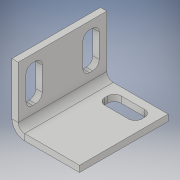
# Autodesk Inventor part: mezzanineBracketRight
Saved by Autodesk Inventor 2017 (Build 210142000, 142)
## iProperties
Created: 2017-03-16
Part Number: mezzanineBracketRight
Material: Generic
Document SubType Name: Sheet Metal
Designer: Zara
Density: 1 g/cm^3
Sheet Metal Rule: Default
Appearance: Default
Author: Zara
Autodesk Inventor part; units mm, degrees
ref_plane "YZ Plane" through (0, 0, 0) normal (1, 0, 0) x (0, 1, 0)
ref_plane "XZ Plane" through (0, 0, 0) normal (0, 1, 0) x (-1, 0, 0)
ref_plane "XY Plane" through (0, 0, 0) normal (0, 0, 1) x (1, 0, 0)
sketch "Sketch1" plane through (0, 0, 0) normal (0, 1, 0) x (-1, 0, 0)
  line L0 (-8.128, 10.6426) -> (8.128, 10.6426)
  line L1 (8.128, 10.6426) -> (8.128, -10.6426)
  line L2 (8.128, -10.6426) -> (-8.128, -10.6426)
  line L3 (-8.128, -10.6426) -> (-8.128, 10.6426)
  line L4 (-8.128, 10.6426) -> (8.128, -10.6426) construction
  line L5 (8.128, 10.6426) -> (-8.128, -10.6426) construction
  point P0 (0, 0)
  dimension "d0" = 21.2852
  dimension "d1" = 16.256
  measures "d0" distance of L0.end L1.end
  measures "d1" distance of L1.end L2.end
extrude "Plate1" add sketch "Sketch1" along normal blind 1.524
sketch "Sketch2" plane through (-6.604, 0, 10.6426) normal (-1, 0, 0) x (0, -1, 0)
  line L0 (0, -21.2852) -> (0, 0)
  line L1 (0, 0) -> (-15.5956, 0)
  line L2 (-15.5956, 0) -> (-15.5956, -21.2852)
  line L3 (-15.5956, -21.2852) -> (0, -21.2852)
  constraints: 6 end point, 1 horizontal, 1 perpendicular, 1 vertical
edge flange "Flange1" height 15.5956 angle 90 thickness 1.524 bend radius 1.524 thickness toward (-1, 0, 0) relief tear relief width 1.524 relief depth 0.762 edges at (-8.128, 1.524, 0) wall of the first edge with corners at (-6.604, 0, -10.6426) (-6.604, 0, 10.6426) (-6.604, 15.5956, 10.6426) (-6.604, 15.5956, -10.6426)
bend "Bend1"
corner "Corner1"
sketch "Sketch3" plane through (-6.604, 15.5956, 10.6426) normal (1, 0, 0) x (0, 0, -1)
  line L0 (0, 0) -> (0, -12.5476) construction
  line L1 (21.2852, -12.5476) -> (21.2852, 0) construction
  circle A0 centre (3.7973, -6.2738) radius 1.5875 construction
  circle A1 centre (17.4879, -6.2738) radius 1.5875 construction
  line L2 (3.7973, -6.2738) -> (17.4879, -6.2738) construction
  line L3 (21.2852, 0) -> (0, 0) construction
  line L4 (10.6426, 0) -> (10.6426, -12.5476) construction
  line L5 (0, -12.5476) -> (21.2852, -12.5476) construction
  line L6 (17.1196, -10.7188) -> (17.8562, -10.7188)
  line L7 (19.4437, -9.1313) -> (19.4437, -3.4163)
  line L8 (17.8562, -1.8288) -> (17.1196, -1.8288)
  line L9 (15.5321, -3.4163) -> (15.5321, -9.1313)
  line L10 (15.5321, -10.7188) -> (19.4437, -1.8288) construction
  line L11 (19.4437, -10.7188) -> (15.5321, -1.8288) construction
  arc A2 (17.1196, -1.8288) -> (15.5321, -3.4163) centre (17.1196, -3.4163) ccw
  arc A3 (19.4437, -3.4163) -> (17.8562, -1.8288) centre (17.8562, -3.4163) ccw
  arc A4 (15.5321, -9.1313) -> (17.1196, -10.7188) centre (17.1196, -9.1313) ccw
  arc A5 (17.8562, -10.7188) -> (19.4437, -9.1313) centre (17.8562, -9.1313) ccw
  line L12 (3.429, -10.7188) -> (4.1656, -10.7188)
  line L13 (5.7531, -9.1313) -> (5.7531, -3.4163)
  line L14 (4.1656, -1.8288) -> (3.429, -1.8288)
  line L15 (1.8415, -3.4163) -> (1.8415, -9.1313)
  line L16 (1.8415, -10.7188) -> (5.7531, -1.8288) construction
  line L17 (5.7531, -10.7188) -> (1.8415, -1.8288) construction
  arc A6 (3.429, -1.8288) -> (1.8415, -3.4163) centre (3.429, -3.4163) ccw
  arc A7 (5.7531, -3.4163) -> (4.1656, -1.8288) centre (4.1656, -3.4163) ccw
  arc A8 (4.1656, -10.7188) -> (5.7531, -9.1313) centre (4.1656, -9.1313) ccw
  arc A9 (1.8415, -9.1313) -> (3.429, -10.7188) centre (3.429, -9.1313) ccw
  point P0 (10.6426, -15.5956)
  point P1 (10.6426, -6.2738)
  dimension "d13" = 13.6906
  dimension "d14" = 3.175
  dimension "d15" = 3.175
  dimension "d16" = 3.9116
  dimension "d17" = 8.89
  dimension "d18" = 1.5875
  dimension "d19" = 3.9116
  dimension "d20" = 8.89
  dimension "d21" = 1.5875
  constraints: 28 end point, 16 point on circle, 16 point on line, 16 tangent, 10 centre point, 8 midpoint, 6 equal radius, 4 parallel, 3 horizontal, 2 perpendicular
  measures "d13" distance of L2.end L2.start
  measures "d14" diameter of A1
  measures "d15" diameter of A0
  measures "d16" distance of L10.start L11.start
  measures "d17" distance of L11.start L10.end
  measures "d18" radius of A2
  measures "d19" distance of L16.start L17.start
  measures "d20" distance of L17.end L16.start
  measures "d21" radius of A6
sketch "Sketch4" plane through (0, 1.524, 0) normal (0, 1, 0) x (1, 0, 0)
  line L0 (-5.08, 10.6426) -> (8.128, 10.6426) construction
  line L1 (4.3815, 4.8768) -> (-1.3335, 4.8768)
  line L2 (-2.921, 6.4643) -> (-2.921, 7.2009)
  line L3 (-1.3335, 8.7884) -> (4.3815, 8.7884)
  line L4 (5.969, 7.2009) -> (5.969, 6.4643)
  arc A0 (-2.921, 6.4643) -> (-1.3335, 4.8768) centre (-1.3335, 6.4643) ccw
  arc A1 (-1.3335, 8.7884) -> (-2.921, 7.2009) centre (-1.3335, 7.2009) ccw
  arc A2 (4.3815, 4.8768) -> (5.969, 6.4643) centre (4.3815, 6.4643) ccw
  arc A3 (5.969, 7.2009) -> (4.3815, 8.7884) centre (4.3815, 7.2009) ccw
  line L5 (8.128, 10.6426) -> (8.128, -10.6426) projected
  line L6 (1.524, 4.8768) -> (1.524, 8.7884) construction
  line L7 (4.3815, -8.7884) -> (-1.3335, -8.7884) construction
  line L8 (-2.921, -7.2009) -> (-2.921, -6.4643) construction
  line L9 (-1.3335, -4.8768) -> (4.3815, -4.8768) construction
  line L10 (5.969, -6.4643) -> (5.969, -7.2009) construction
  arc A4 (-2.921, -7.2009) -> (-1.3335, -8.7884) centre (-1.3335, -7.2009) ccw construction
  arc A5 (-1.3335, -4.8768) -> (-2.921, -6.4643) centre (-1.3335, -6.4643) ccw construction
  arc A6 (4.3815, -8.7884) -> (5.969, -7.2009) centre (4.3815, -7.2009) ccw construction
  arc A7 (5.969, -6.4643) -> (4.3815, -4.8768) centre (4.3815, -6.4643) ccw construction
  line L11 (1.524, -8.7884) -> (1.524, -4.8768) construction
  line L12 (8.128, -10.6426) -> (-5.08, -10.6426) construction
  point P0 (0, 0)
  point P1 (1.524, 6.8326)
  point P2 (1.524, -6.8326)
  dimension "d26" = 1.5875
  dimension "d32" = 3.9116
  dimension "d33" = 8.89
  dimension "d34" = 6.604
  dimension "d35" = 3.81
  dimension "d36" = 1.5875
  dimension "d37" = 3.9116
  dimension "d38" = 8.89
  dimension "d39" = 3.81
  dimension "d40" = 6.604
  constraints: 20 end point, 16 point on circle, 16 tangent, 8 centre point, 6 equal radius, 6 midpoint, 4 parallel, 2 horizontal, 2 perpendicular, 2 vertical
  measures "d26" radius of A0
  measures "d32" distance between parallel lines of L3 L1
  measures "d33" distance between parallel lines of L2 L4
  measures "d34" distance between parallel lines of L6 L5
  measures "d35" distance from line of point (1.524, 6.833) L0
  measures "d36" radius of A4
  measures "d37" distance between parallel lines of L9 L7
  measures "d38" distance between parallel lines of L8 L10
  measures "d39" distance from line of L12 point (1.524, -6.833)
  measures "d40" distance from line of point (1.524, -6.833) L5
extrude "Extrusion1" cut sketch "Sketch3" against normal through all
extrude "Extrusion3" cut sketch "Sketch4" against normal through all
equation "\"d3\" = BendReliefWidth"
equation "\"d4\" = BendReliefDepth"
equation "\"d5\" = MinimumRemnant"
equation "\"d6\" = BendRadius"
equation "\"d9\" = BendRadius"
equation "\"d10\" = CornerReliefSize"
equation "\"d11\" = GapSize"
equation "\"d12\" = JacobiRadiusSize"
equation "\"BendRadius\" = Thickness"
equation "\"BendReliefWidth\" = Thickness"
equation "\"BendReliefDepth\" = 0.5 * Thickness"
equation "\"CornerReliefSize\" = 4 * Thickness"
equation "\"MinimumRemnant\" = 2 * Thickness"
equation "\"TransitionRadius\" = BendRadius"
equation "\"JacobiRadiusSize\" = BendRadius"
equation "\"GapSize\" = Thickness"
equation "\"d2\" = BendRadius"
equation "\"Thickness\" = 1.524"
body "Solid1"
